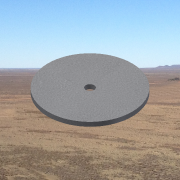
# Autodesk Inventor part: 2f1abs
Saved by Autodesk Inventor 2013 SP2 (Build 170200200, 200)
## iProperties
Company: HERA Project
Created: 2013-06-03
Part Number: 2f1abs
Material: GFRC
Document SubType Name: Modeling
Designer: David DeBoer
Density: 1.7 g/cm^3
Description: Feed absorbing disk
Mass: 1083.04 g
Surface Area: 1114.76 cm^2
Volume: 637.083 cm^3
Author: David DeBoer
Title: Feed absorbing disk
Autodesk Inventor part; units mm, degrees
ref_plane "YZ Plane" through (0, 0, 0) normal (1, 0, 0) x (0, 1, 0)
ref_plane "XZ Plane" through (0, 0, 0) normal (0, 1, 0) x (-1, 0, 0)
ref_plane "XY Plane" through (0, 0, 0) normal (0, 0, 1) x (1, 0, 0)
sketch "Sketch1" plane through (0, 0, 0) normal (0, 1, 0) x (-1, 0, 0)
  circle A0 centre (0, 0) radius 127
  circle A1 centre (0, 0) radius 12.7
  dimension "d0" = 254
  dimension "d2" = 25.4
  constraints: 2 centre point, 2 coincident
  measures "d0" diameter of A0
  measures "d2" diameter of A1
extrude "Extrusion1" add sketch "Sketch1" along normal blind 12.7
body "Solid1"
